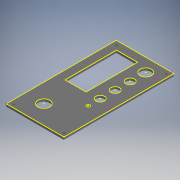
# Autodesk Inventor part: component box cover
Saved by Autodesk Inventor 2021 (Build 250183000, 183)
## iProperties
Created: 2023-01-12
Part Number: component box cover
Material: Generic
Document SubType Name: Modeling
Designer: boyle
Density: 1 g/cm^3
Appearance: Default
Author: boyle
Autodesk Inventor part; units mm, degrees
ref_plane "YZ Plane" through (0, 0, 0) normal (1, 0, 0) x (0, 1, 0)
ref_plane "XZ Plane" through (0, 0, 0) normal (0, 1, 0) x (-1, 0, 0)
ref_plane "XY Plane" through (0, 0, 0) normal (0, 0, 1) x (1, 0, 0)
sketch "Sketch1" plane through (0, 0, 0) normal (0, 1, 0) x (-1, 0, 0)
  line L0 (0, 0) -> (-111.76, 0)
  line L1 (-111.76, 0) -> (-111.76, 213.36)
  line L2 (-111.76, 213.36) -> (0, 213.36)
  line L3 (0, 213.36) -> (0, 0)
  line L4 (-111.76, 212.09) -> (-111.76, 0) projected
  line L5 (0, 212.09) -> (-111.76, 212.09) projected
  line L6 (0, 0) -> (0, 212.09) projected
  line L7 (-111.76, 0) -> (0, 0) projected
  line L8 (-111.76, 0) -> (0, 0) projected
  line L9 (0, 0) -> (0, 212.09) projected
  line L10 (-111.76, 212.09) -> (-111.76, 0) projected
  line L11 (-111.76, 0) -> (0, 0) projected
  line L12 (0, 218.44) -> (-107.95, 218.44) projected
  line L13 (-107.95, 218.44) -> (-107.95, 212.09) projected
  line L14 (0, 212.09) -> (0, 218.44) projected
  dimension "d0" = 111.76
  dimension "d1" = 213.36
  constraints: 8 end point, 2 parallel, 1 horizontal, 1 perpendicular
  measures "d0" distance of L1.end L2.end
  measures "d1" distance of L0.end L1.end
extrude "Extrusion1" add sketch "Sketch1" along normal blind 4.826 contours L0 L1 L5 L3 | L5 L13 L2 L3 | L1 L2 L13 L5
sketch "Sketch2" plane through (0, 4.826, 0) normal (0, 1, 0) x (1, 0, 0)
  line L0 (111.76, 0) -> (0, 0) projected
  line L1 (0, 0) -> (0, -213.36) projected
  line L2 (88.8491, -51.3544) -> (82.4991, -51.3544)
  line L3 (82.4991, -51.3544) -> (82.4991, -0.0669)
  line L4 (82.4991, -0.0669) -> (82.4991, -12.7669)
  line L5 (82.4991, -0.0669) -> (82.4991, -25.4669)
  circle A0 centre (82.4991, -25.4669) radius 11
  line L6 (82.4991, -25.4669) -> (82.4991, -51.8669)
  line L7 (82.4991, -36.4669) -> (82.4991, -61.8669)
  circle A1 centre (82.4928, -55.6695) radius 8.25
  line L8 (82.4991, -48.0194) -> (82.4991, -56.1194)
  line L9 (82.4928, -63.9195) -> (82.4928, -84.7195)
  circle A2 centre (82.4928, -84.7195) radius 8.25
  line L10 (82.4928, -92.9695) -> (82.4928, -113.7721)
  circle A3 centre (82.4928, -113.7721) radius 8.25
  circle A4 centre (36.0751, -176.7145) radius 11.5
  line L11 (10.6751, -176.7232) -> (36.0751, -176.7232)
  line L12 (57.6456, -16.3037) -> (16.6456, -16.3037)
  line L13 (16.6456, -16.3037) -> (16.6456, -116.3037)
  line L14 (16.6456, -116.3037) -> (57.6456, -116.3037)
  line L15 (57.6456, -116.3037) -> (57.6456, -16.3037)
  line L16 (36.0751, -176.7232) -> (36.0751, -151.3232)
  line L17 (82.8401, -122.0148) -> (82.8401, -137.2548)
  circle A5 centre (82.8401, -137.2548) radius 3.25
  line L18 (0, -213.36) -> (111.76, -213.36) projected
  line L19 (111.76, -213.36) -> (111.76, 0) projected
  dimension "d14" = 22
  dimension "d18" = 16.5
  dimension "d13" = 25.4
  dimension "d17" = 25.4
  dimension "d19" = 8.1
  dimension "d20" = 20.8
  dimension "d22" = 20.8026
  dimension "d24" = 23
  dimension "d27" = 25.4
  dimension "d28" = 41
  dimension "d29" = 100
  dimension "d30" = 25.4
  dimension "d31" = 15.24
  dimension "d32" = 6.5
  constraints: 32 end point, 4 coincident, 3 point on line, 3 vertical alignment, 2 centre point, 2 parallel, 2 perpendicular, 1 horizontal, 1 vertical, 9 other
  measures "d13" distance of L3.end L5.end
  measures "d17" distance of L7.end L7.start
  measures "d19" distance of L8.start L8.end
  measures "d20" distance of L9.start L9.end
  measures "d22" distance of L10.start L10.end
  measures "d24" diameter of A4
  measures "d27" distance of L11.start L11.end
  measures "d28" distance of L14.end L13.end
  measures "d29" distance of L13.end L12.end
  measures "d30" distance of L11.end L16.end
  measures "d31" distance of L17.start L17.end
  measures "d32" diameter of A5
extrude "Extrusion3" cut sketch "Sketch2" against normal blind 25.4 contours A0 L3 | A5 | A3 | A2 | A1 | L3 A0 | A4 L11 L16 | L16 L11 A4 | L15 L14 L13 L12
sketch "Sketch3" plane through (0, 4.826, 0) normal (0, 1, 0) x (1, 0, 0)
  circle A0 centre (82.4991, -25.4669) radius 11 projected
  circle A1 centre (82.4928, -113.7721) radius 8.25 projected
  line L0 (57.6456, -116.3037) -> (16.6456, -116.3037) projected
  line L1 (16.6456, -116.3037) -> (16.6456, -16.3037) projected
  line L2 (16.6456, -16.3037) -> (57.6456, -16.3037) projected
  line L3 (57.6456, -16.3037) -> (57.6456, -116.3037) projected
  circle A2 centre (82.4928, -55.6695) radius 8.25 projected
  circle A3 centre (82.4928, -84.7195) radius 8.25 projected
  line L4 (111.76, 0) -> (0, 0) projected
  line L5 (0, 0) -> (0, -213.36) projected
  circle A4 centre (36.0751, -176.7145) radius 11.5 projected
  line L6 (57.6456, -116.3037) -> (16.6456, -116.3037) projected
  line L7 (16.6456, -116.3037) -> (16.6456, -16.3037) projected
  line L8 (16.6456, -16.3037) -> (57.6456, -16.3037) projected
  circle A5 centre (82.8401, -137.2548) radius 3.25 projected
  line L9 (111.76, 0) -> (0, 0) projected
  line L10 (0, 0) -> (0, -213.36) projected
  line L11 (0, 0) -> (0, -213.36) projected
  circle A6 centre (36.0751, -176.7145) radius 11.5 projected
  circle A7 centre (82.8401, -137.2548) radius 3.25 projected
  line L12 (57.6456, -16.3037) -> (57.6456, -116.3037) projected
  line L13 (0, -213.36) -> (111.76, -213.36) projected
  line L14 (111.76, -213.36) -> (111.76, 0) projected
  point P0 (107.95, -122.8721)
  point P1 (107.95, -24.8721)
  point P2 (107.95, 0)
  constraints: 2 other
sketch "Sketch5" plane through (0, 4.826, 0) normal (0, 1, 0) x (1, 0, 0)
  line L0 (0, 0) -> (0, -213.36) projected
  line L1 (0, -213.36) -> (0, -208.36)
  circle A0 centre (8.81, -8.81) radius 2 projected
  circle A1 centre (8.81, -207.09) radius 2 projected
  circle A2 centre (105.49, -207.09) radius 2 projected
  circle A3 centre (105.49, -8.81) radius 2 projected
  circle A4 centre (105.49, -8.81) radius 2
  circle A5 centre (105.49, -207.09) radius 2
  circle A6 centre (8.81, -207.09) radius 2
  circle A7 centre (8.81, -8.81) radius 2
  dimension "d36" = 5
  constraints: 4 centre point, 4 coincident, 4 concentric, 2 end point, 1 point on line
  measures "d36" distance of L0.end L1.end
extrude "Extrusion5" cut sketch "Sketch5" against normal up to next
body "Solid1"
